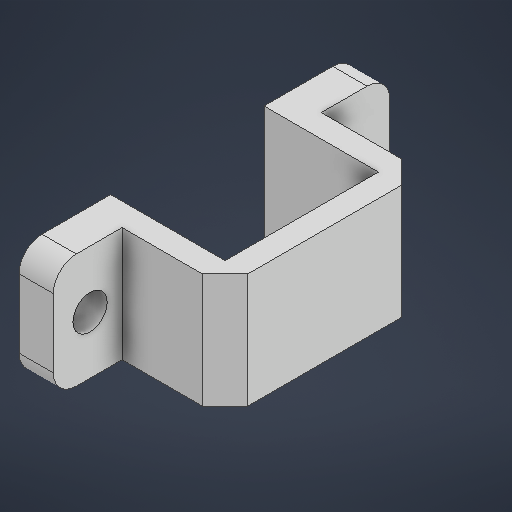
# Autodesk Inventor part: silnik_lockedin
Saved by Autodesk Inventor 2027 (Build 310192060, 192F)
## iProperties
Created: 2026-05-29
Part Number: silnik_lockedin
Material: Ogólny
Document SubType Name: Modeling
Designer: User
Density: 1 g/cm^3
Appearance: Domyślna
Author: User
Autodesk Inventor part; units mm, degrees
ref_plane "YZ Plane" through (0, 0, 0) normal (1, 0, 0) x (0, 1, 0)
ref_plane "XZ Plane" through (0, 0, 0) normal (0, 1, 0) x (-1, 0, 0)
ref_plane "XY Plane" through (0, 0, 0) normal (0, 0, 1) x (1, 0, 0)
sketch "Szkic1" plane through (0, 0, 0) normal (0, 1, 0) x (-1, 0, 0)
  line L0 (-4, 6.5) -> (4, 6.5) construction
  line L1 (4, 6.5) -> (4, -6.5) construction
  line L2 (4, -6.5) -> (-4, -6.5) construction
  line L3 (-4, -6.5) -> (-4, 6.5) construction
  line L4 (-4, 6.5) -> (4, -6.5) construction
  line L5 (4, 6.5) -> (-4, -6.5) construction
  line L6 (-5, -6.7) -> (5, -6.7)
  line L7 (5, -6.7) -> (5, 6.7)
  line L8 (5, 6.7) -> (-5, 6.7)
  line L9 (-5, 6.7) -> (-5, -6.7)
  line L10 (-5, -6.7) -> (5, 6.7) construction
  line L11 (5, -6.7) -> (-5, 6.7) construction
  line L12 (5, 6.7) -> (5, 11.7)
  line L13 (5, -6.7) -> (5, -11.7)
  line L14 (5, 11.7) -> (5, 14.7)
  line L15 (5, -11.7) -> (5, -14.7)
  line L16 (5, 14.7) -> (2, 14.7)
  line L17 (2, 14.7) -> (2, 11.7)
  line L18 (2, 11.7) -> (5, 11.7)
  line L19 (5, 11.7) -> (5, 14.7)
  line L20 (5, -14.7) -> (2, -14.7)
  line L21 (2, -14.7) -> (2, -11.7)
  line L22 (2, -11.7) -> (5, -11.7)
  line L23 (5, -11.7) -> (5, -14.7)
  line L24 (-5, 0) -> (-7, 0)
  line L25 (-5, 6.7) -> (-7, 6.7)
  line L26 (-5, -6.7) -> (-7, -6.7)
  line L27 (2, 11.7) -> (2, 8.7)
  line L28 (-7, 6.7) -> (-7, 0)
  line L29 (-7, 0) -> (-7, -6.7)
  line L30 (2, -11.7) -> (2, -8.7)
  line L31 (-5, 6.7) -> (-5, 8.7)
  line L32 (-5, 8.7) -> (2, 8.7)
  line L33 (-5, -6.7) -> (-5, -8.7)
  line L34 (-5, -8.7) -> (2, -8.7)
  line L35 (-5, 8.7) -> (-7, 6.7)
  line L36 (-7, -6.7) -> (-5, -8.7)
  point P0 (0, 0)
  dimension "d0" = 8
  dimension "d1" = 13
  dimension "d2" = 10
  dimension "d3" = 13.4
  dimension "d4" = 5
  dimension "d5" = 5
  dimension "d6" = 3
  dimension "d7" = 3
  dimension "d8" = 3
  dimension "d9" = 3
  dimension "d10" = 2
  dimension "d11" = 2
  dimension "d12" = 2
  dimension "d13" = 3
  dimension "d14" = 3
  dimension "d15" = 2
  dimension "d16" = 2
  constraints: 74 end point, 8 parallel, 7 horizontal, 7 vertical, 5 midpoint, 5 perpendicular
  measures "d0" distance of L1.end L2.end
  measures "d1" distance of L0.end L1.end
  measures "d2" distance of L8.end L7.end
  measures "d3" distance of L7.end L6.end
  measures "d4" distance of L7.end L12.end
  measures "d5" distance of L6.end L13.end
  measures "d6" distance of L12.end L14.end
  measures "d7" distance of L13.end L15.end
  measures "d8" distance of L18.end L17.end
  measures "d9" distance of L21.end L22.end
  measures "d10" distance of L24.start L24.end
  measures "d11" distance of L8.end L25.end
  measures "d12" distance of L6.start L26.end
  measures "d13" distance of L17.end L27.end
  measures "d14" distance of L21.end L30.end
  measures "d15" distance of L8.end L31.end
  measures "d16" distance of L6.start L33.end
extrude "Wyciągnięcie proste1" add sketch "Szkic1" along normal blind 10 contours L26 L29 L24 L9 | L33 L36 L26 | L6 L13 L22 L30 L34 L33 | L24 L28 L25 L9 | L8 L31 L32 L27 L18 L12 | L15 L20 L21 L22 | L25 L35 L31 | L18 L17 L16 L14
sketch "Szkic2" plane through (-2, 0, 14.7) normal (1, 0, 0) x (0, 0, -1)
  line L0 (0, 10) -> (6, 10) construction
  line L1 (6, 0) -> (6, 10) construction
  line L2 (0, 0) -> (0, 10) construction
  line L3 (6, 0) -> (0, 0) construction
  line L4 (14.7, 0) -> (14.7, 10) construction
  line L5 (8, 10) -> (21.4, 10) construction
  circle A0 centre (3.2, 5) radius 1.5
  circle A1 centre (26.2, 5) radius 1.5
  line L6 (23.4, 0) -> (23.4, 10) projected
  line L7 (0, 0) -> (6, 10) construction
  line L8 (6, 0) -> (0, 10) construction
  line L9 (6, 0) -> (6, 10) projected
  point P0 (6, 5)
  point P1 (6, 5)
  dimension "d19" = 3
  dimension "d27" = 2.8
  dimension "d28" = 5
  constraints: 8 end point, 3 midpoint, 2 centre point, 1 perpendicular, 1 symmetric about line, 1 other
  measures "d19" diameter of A0
  measures "d27" distance of A0.centre point (6, 5)
  measures "d28" distance from line of L0 A0.centre
extrude "Wyciągnięcie proste2" cut sketch "Szkic2" against normal blind 6.65
fillet "Zaokrąglenie1" radius 2 4 edges at (-3.5, 10, 14.7) (-3.5, 0, 14.7) (-3.5, 10, -14.7) (-3.5, 0, -14.7)
